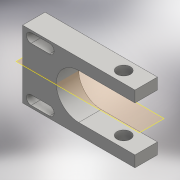
# Autodesk Inventor part: Y-pulley-mount
Saved by Autodesk Inventor 2016 (Build 200138000, 138)
## iProperties
Created: 2015-05-19
Part Number: Y-pulley-mount
Material: Generic
Document SubType Name: Modeling
Designer: as
Mass: 7.21001 g
Surface Area: 43.7372 cm^2
Volume: 7.21001 cm^3
Density: 1 g/cm^3
Appearance: Default
Author: as
Autodesk Inventor part; units mm, degrees
ref_plane "YZ Plane" through (0, 0, 0) normal (1, 0, 0) x (0, 1, 0)
ref_plane "XZ Plane" through (0, 0, 0) normal (0, 1, 0) x (-1, 0, 0)
ref_plane "XY Plane" through (0, 0, 0) normal (0, 0, 1) x (1, 0, 0)
sketch "Sketch1" plane through (0, 0, 0) normal (0, 0, 1) x (1, 0, 0)
  line L0 (0, 0) -> (-50, 0)
  line L1 (-50, 0) -> (-50, -10)
  line L2 (-50, -10) -> (0, -10)
  line L3 (0, -10) -> (0, 0)
  circle A0 centre (-10, -5) radius 3
  dimension "d0" = 50
  dimension "d1" = 6
  constraints: 8 end point, 2 parallel, 1 centre point, 1 horizontal, 1 perpendicular
  measures "d0" distance of L2.end L1.end
  measures "d1" diameter of A0
extrude "Extrusion1" add sketch "Sketch1" along normal blind 30
sketch "Sketch2" plane through (-50, -10, 0) normal (0, -1, 0) x (1, 0, 0)
  line L0 (50, 0) -> (50, 30) projected
  line L1 (50, 15) -> (25, 15) construction
  line L2 (50, 25) -> (25, 25)
  line L3 (25, 5) -> (50, 5)
  arc A0 (50, 5) -> (50, 25) centre (50, 15) ccw
  arc A1 (25, 25) -> (25, 5) centre (25, 15) ccw
  line L4 (0, 0) -> (50, 0) projected
  point P0 (37.5, 15)
  dimension "d4" = 25
  dimension "d5" = 20
  dimension "d6" = 15
  constraints: 8 end point, 4 point on circle, 4 tangent, 2 centre point, 2 midpoint, 1 horizontal, 1 parallel
  measures "d4" distance of L1.start L1.end
  measures "d5" diameter of A1
  measures "d6" distance between parallel lines of L4 L1
extrude "Extrusion2" cut sketch "Sketch2" against normal through all
sketch "Sketch3" plane through (-50, 0, 0) normal (0, 1, 0) x (1, 0, 0)
  line L0 (1.75, -3.05) -> (14.05, -3.05) construction
  line L1 (3.8, -5.1) -> (12, -5.1)
  line L2 (12, -1) -> (3.8, -1)
  arc A0 (3.8, -1) -> (3.8, -5.1) centre (3.8, -3.05) ccw
  arc A1 (12, -5.1) -> (12, -1) centre (12, -3.05) ccw
  line L3 (0, 0) -> (50, 0) projected
  point P0 (7.9, -3.05)
  dimension "d9" = 4.1
  dimension "d10" = 1
  constraints: 8 end point, 6 point on circle, 4 tangent, 2 centre point, 2 point on line, 1 horizontal, 1 midpoint, 1 parallel
  measures "d9" diameter of A1
  measures "d10" distance between parallel lines of L3 L2
extrude "Extrusion3" cut sketch "Sketch3" against normal through all
ref_plane "Work Plane1" through (0, 0, 15) normal (0, 0, 1) x (1, 0, 0)
mirror "Mirror1" about plane through (0, 0, 15) normal (0, 0, 1) of "Extrusion3"
equation "\"d6\" = 0.5 * d2"
equation "\"d13\" = -0.5 * d2"
equation "\"d2\" = 30"
body "Solid1"
